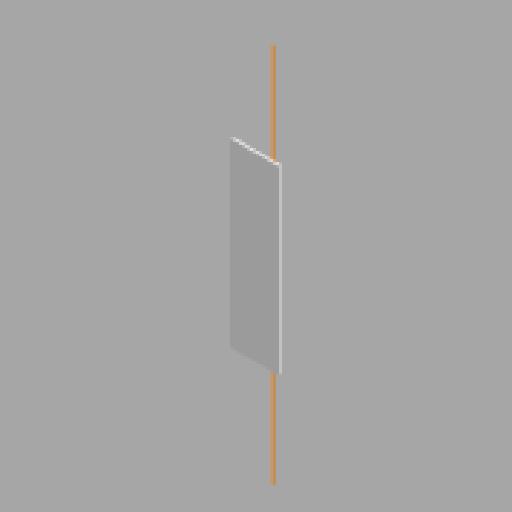
# Autodesk Inventor part: Порог_Левый
Saved by Autodesk Inventor 2025 (Build 290162000, 162)
## iProperties
Created: 2025-04-24
Part Number: Порог_Левый
Material: Типовые
Document SubType Name: Modeling
Designer: Artem Sannikov
Density: 1 g/cm^3
Appearance: По умолчанию
Author: Artem Sannikov
Autodesk Inventor part; units mm, degrees
ref_plane "YZ Plane" through (0, 0, 0) normal (1, 0, 0) x (0, 1, 0)
ref_plane "XZ Plane" through (0, 0, 0) normal (0, 1, 0) x (-1, 0, 0)
ref_plane "XY Plane" through (0, 0, 0) normal (0, 0, 1) x (1, 0, 0)
ref_plane "РабПлоскость1" through (0, 0, 0) normal (0, 0, 1) x (1, 0, 0)
sketch "Эскиз1" plane through (0, 0, 0) normal (0, 0, 1) x (1, 0, 0)
  line L0 (-41.5, 251.765) -> (-1.5, 251.765) construction
  line L1 (-41.5, 258.235) -> (-1.5, 258.235) construction
  line L2 (-41.5, 245) -> (-1.5, 245) construction
  line L3 (-41.5, 265) -> (-1.5, 265) construction
  line L4 (-21.5, 265) -> (-21.5, 245) construction
  line L5 (-55.5, 383.1594) -> (12.5, 383.1594)
  line L6 (12.5, 383.1594) -> (12.5, 126.8406)
  line L7 (12.5, 126.8406) -> (-55.5, 126.8406)
  line L8 (-55.5, 126.8406) -> (-55.5, 383.1594)
  line L9 (-55.5, 383.1594) -> (12.5, 126.8406) construction
  line L10 (12.5, 383.1594) -> (-55.5, 126.8406) construction
  point P0 (0, 0)
  point P1 (-21.5, 255)
  constraints: 14 end point, 5 midpoint, 2 parallel, 1 horizontal, 1 perpendicular, 1 other
extrude "Выдавливание1" add sketch "Эскиз1" along normal blind 4
sketch "Эскиз2" plane through (-55.5, 126.8406, 0) normal (0, -1, 0) x (1, 0, 0)
  line L0 (68, 0) -> (68, 24.2132) projected
  line L1 (0, 4) -> (68, 4) projected
  line L2 (38, 24.2132) -> (-8, 0) projected
  line L3 (68, 24.2132) -> (38, 24.2132) projected
  line L4 (68, 24.2132) -> (38, 24.2132) projected
  line L5 (68, 0) -> (68, 24.2132) projected
  line L6 (68, 0) -> (-8, 0) projected
  line L7 (38, 24.2132) -> (-8, 0) projected
  point P0 (55.5, 0)
extrude "Выдавливание2" add sketch "Эскиз2" against normal blind 1.5
sketch "Эскиз3" plane through (-55.5, 128.3406, 0) normal (-1, 0, 0) x (0, 0, 1)
  line L0 (0, 0) -> (4, 0) projected
  line L1 (4, 254.8188) -> (4, 0) projected
  line L2 (0, 254.8188) -> (4, 254.8188) projected
  line L3 (0, 254.8188) -> (0, 0) projected
  point P0 (0, -128.3406)
extrude "Выдавливание3" add sketch "Эскиз3" along normal up to surface (8 mm away)
ref_plane "РабПлоскость2" through (-55.5, 255.75, 0) normal (0, 1, 0) x (1, 0, 0)
